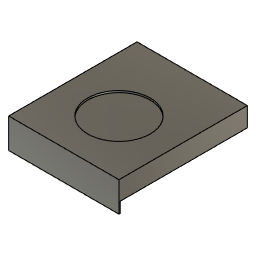
slider (Autodesk Fusion 360 design; units mm, degrees)
Autodesk Fusion 360 part; units mm, degrees
note: some values were not read from the file. Set by a fixed rule: which sketch regions a step uses.
sketch "Sketch1" plane through (0, 0, 0) normal (0, 0, 1) x (1, 0, 0) in component "Gerüst"
  line L0 (0, 0) -> (114, 0)
  line L1 (114, 0) -> (114, 114)
  line L2 (114, 114) -> (0, 114)
  line L3 (0, 114) -> (0, 0)
  circle A0 centre (7.25, 6.75) radius 2.75
  line L4 (57, 114) -> (57, 0) construction
  line L5 (0, 57) -> (114, 57) construction
  circle A1 centre (7.25, 35.25) radius 2.75
  circle A2 centre (28.75, 6.75) radius 2.75
  circle A3 centre (106.75, 6.75) radius 2.75
  circle A4 centre (85.25, 6.75) radius 2.75
  circle A5 centre (106.75, 35.25) radius 2.75
  circle A6 centre (7.25, 78.75) radius 2.75
  circle A7 centre (7.25, 107.25) radius 2.75
  circle A8 centre (28.75, 107.25) radius 2.75
  circle A9 centre (85.25, 107.25) radius 2.75
  circle A10 centre (106.75, 107.25) radius 2.75
  circle A11 centre (106.75, 78.75) radius 2.75
  line L6 (21, 100.5) -> (93, 100.5)
  line L7 (93, 100.5) -> (93, 13.5)
  line L8 (93, 13.5) -> (21, 13.5)
  line L9 (21, 13.5) -> (21, 100.5)
  line L10 (37, 114) -> (37, 131)
  line L11 (37, 131) -> (77, 131)
  line L12 (77, 131) -> (77, 114)
  line L13 (57, 131) -> (57, 114) construction
  line L14 (21, 64.5) -> (93, 64.5)
  line L15 (93, 64.5) -> (93, 49.5)
  line L16 (93, 49.5) -> (21, 49.5)
  line L17 (21, 49.5) -> (21, 64.5)
  line L18 (21, 64.5) -> (93, 49.5) construction
  line L19 (93, 64.5) -> (21, 49.5) construction
  point P0 (57, 57)
  dimension "d1" = 114
  dimension "d2" = 114
  dimension "d3" = 5.5
  dimension "d5" = 4.5
  dimension "d6" = 4
  dimension "d7" = 23
  dimension "d8" = 16
  dimension "d9" = 11
  dimension "d10" = 11
  dimension "d11" = 4
  dimension "d12" = 4
  dimension "d15" = 40
  dimension "d16" = 17
  dimension "d61" = 15
  constraint horizontal L0
  constraint vertical L1
  constraint horizontal L2
  constraint vertical L3
  constraint coincident L0.start L3.end
  constraint midpoint L2 L4.start
  constraint midpoint L0 L4.end
  constraint midpoint L3 L5.start
  constraint midpoint L1 L5.end
  constraint equal A0 A1
  constraint vertical A0.centre A1.centre
  constraint horizontal A0.centre A2.centre
  constraint equal A0 A2
  constraint symmetric A0 L4 A3
  constraint symmetric L4 A1 A5
  constraint symmetric L4 A2 A4
  constraint symmetric A0 L5 A7
  constraint symmetric L5 A1 A6
  constraint symmetric L5 A2 A8
  constraint symmetric L5 A3 A10
  constraint symmetric L5 A4 A9
  constraint symmetric L5 A5 A11
  constraint horizontal L6
  constraint vertical L7
  constraint horizontal L8
  constraint vertical L9
  constraint coincident L2 L10.start
  constraint parallel L2 L11
  constraint coincident L2 L12.end
  constraint midpoint L11 L13.start
  constraint coincident L2 L4.start
  constraint perpendicular L2 L13
  constraint collinear L4 L13
  constraint perpendicular L11 L12
  constraint perpendicular L10 L11
  constraint perpendicular L14 L15
  constraint parallel L14 L16
  constraint parallel L15 L17
  constraint horizontal L14
  constraint coincident L9 L14.start
  constraint coincident L18 P0
  constraint coincident L19 P0
  constraint midpoint L4 P0
  measures "d1" distance of L0.start L2.end
  measures "d2" distance of L0.start L0.end
  measures "d3" diameter of A0
  measures "d5" distance of L3 A0
  measures "d6" distance of L0 A0
  measures "d7" distance of A0 A1
  measures "d8" distance of A0 A2
  measures "d9" distance of A7 L9
  measures "d10" distance of A10 L7
  measures "d11" distance of A7 L6
  measures "d12" distance of A0 L8
  measures "d15" distance of L10.end L11.end
  measures "d16" distance of L2 L11
  measures "d61" distance of L14 L16
extrude "Extrude1" add sketch "Sketch1" along normal blind 5 makes body 1 in component "Gerüst"
sketch "Sketch8" plane through (0, 0, 0) normal (0, 0, -1) x (1, 0, 0) in component "Gerüst"
  circle A0 centre (106.75, -107.25) radius 2.75
  line L0 (21, -13.5) -> (93, -13.5)
  line L1 (93, -13.5) -> (93, -100.5)
  line L2 (93, -100.5) -> (21, -100.5)
  line L3 (21, -100.5) -> (21, -13.5)
  circle A1 centre (28.75, -107.25) radius 2.75
  circle A2 centre (85.25, -107.25) radius 2.75
  circle A3 centre (7.25, -107.25) radius 2.75
  circle A4 centre (85.25, -6.75) radius 2.75
  circle A5 centre (106.75, -78.75) radius 2.75
  circle A6 centre (106.75, -6.75) radius 2.75
  circle A7 centre (7.25, -78.75) radius 2.75
  circle A8 centre (28.75, -6.75) radius 2.75
  circle A9 centre (7.25, -35.25) radius 2.75
  circle A10 centre (106.75, -35.25) radius 2.75
  circle A11 centre (7.25, -6.75) radius 2.75
  line L4 (0, -114) -> (37, -114)
  line L5 (37, -114) -> (37, -131)
  line L6 (37, -131) -> (77, -131)
  line L7 (77, -131) -> (77, -114)
  line L8 (77, -114) -> (114, -114)
  line L9 (114, -114) -> (114, 0)
  line L10 (114, 0) -> (0, 0)
  line L11 (0, 0) -> (0, -114)
  line L12 (37, -131) -> (77, -131)
  line L13 (77, -131) -> (77, -117)
  line L14 (77, -117) -> (37, -117)
  line L15 (37, -117) -> (37, -131)
  dimension "d30" = 14
  constraint horizontal L12
  constraint vertical L13
  constraint horizontal L14
  constraint vertical L15
  constraint coincident L7 L13.end
  constraint coincident L5.end L6.start
  measures "d30" distance of L6.end L13.end
extrude "Extrude3" add sketch "Sketch8" along normal blind 29 contours L5 L6 L7 L12 L13 L14 L15 bodies 1 in component "Gerüst"
sketch "Sketch9" plane through (0, 0, -29) normal (0, 0, -1) x (1, 0, 0) in component "Gerüst"
  line L0 (37, -117) -> (37, -131)
  line L1 (37, -131) -> (77, -131)
  line L2 (77, -131) -> (77, -117)
  line L3 (77, -117) -> (37, -117)
  line L4 (37, -119) -> (77, -119)
  line L5 (77, -119) -> (77, -129)
  line L6 (77, -129) -> (37, -129)
  line L7 (37, -129) -> (37, -119)
  dimension "d33" = 2
  dimension "d34" = 2
  constraint horizontal L4
  constraint vertical L5
  constraint horizontal L6
  constraint vertical L7
  constraint coincident L2 L5.end
  constraint coincident L0 L4.start
  measures "d33" distance of L3 L4
  measures "d34" distance of L1 L6
extrude "Extrude4" cut sketch "Sketch9" against normal blind 6 contours L0 L2 L4 L5 L6 L7 bodies 1 in component "Gerüst"
sketch "Sketch10" plane through (0, 0, 5) normal (0, 0, 1) x (-1, 0, 0) in component "Gerüst"
  circle A0 centre (-106.75, -107.25) radius 2.75
  circle A1 centre (-85.25, -6.75) radius 2.75
  circle A2 centre (-106.75, -78.75) radius 2.75
  circle A3 centre (-7.25, -78.75) radius 2.75
  circle A4 centre (-7.25, -107.25) radius 2.75
  circle A5 centre (-28.75, -107.25) radius 2.75
  line L0 (-93, -13.5) -> (-21, -13.5)
  line L1 (-21, -13.5) -> (-21, -100.5)
  line L2 (-21, -100.5) -> (-93, -100.5)
  line L3 (-93, -100.5) -> (-93, -13.5)
  circle A6 centre (-7.25, -35.25) radius 2.75
  circle A7 centre (-85.25, -107.25) radius 2.75
  circle A8 centre (-106.75, -35.25) radius 2.75
  circle A9 centre (-28.75, -6.75) radius 2.75
  circle A10 centre (-106.75, -6.75) radius 2.75
  circle A11 centre (-7.25, -6.75) radius 2.75
  line L4 (-37, -114) -> (0, -114)
  line L5 (0, -114) -> (0, 0)
  line L6 (0, 0) -> (-114, 0)
  line L7 (-114, 0) -> (-114, -114)
  line L8 (-114, -114) -> (-77, -114)
  line L9 (-77, -114) -> (-77, -131)
  line L10 (-77, -131) -> (-37, -131)
  line L11 (-37, -131) -> (-37, -114)
  line L12 (-41, -131) -> (-73, -131)
  line L13 (-73, -131) -> (-73, -119)
  line L14 (-73, -119) -> (-41, -119)
  line L15 (-41, -119) -> (-41, -131)
  line L16 (-114, -114) -> (0, -114)
  line L17 (-77, -131) -> (-77, -114)
  line L18 (-37, -114) -> (-37, -131)
  dimension "d38" = 4
  dimension "d39" = 4
  dimension "d40" = 12
  constraint horizontal L12
  constraint vertical L13
  constraint horizontal L14
  constraint vertical L15
  constraint coincident L10 L12.start
  measures "d38" distance of L13 L17
  measures "d39" distance of L15 L18
  measures "d40" distance of L12.end L13.end
extrude "Extrude5" cut sketch "Sketch10" against normal up to surface (25 mm away) contours L10 L12 L13 L14 L15 bodies 1 in component "Gerüst"
sketch "Sketch11" plane through (0, 0, -23) normal (0, 0, -1) x (1, 0, 0) in component "Gerüst"
  line L0 (37, -129) -> (77, -129)
  line L1 (77, -129) -> (77, -119)
  line L2 (77, -119) -> (37, -119)
  line L3 (37, -119) -> (37, -129)
  circle A0 centre (57, -124) radius 1.75
  dimension "d44" = 3.5
  dimension "d45" = 5
  dimension "d46" = 20
  measures "d44" diameter of A0
  measures "d45" distance of L2 A0.centre
  measures "d46" distance of L3 A0.centre
extrude "Extrude6" cut sketch "Sketch11" against normal up to surface (3 mm away) contours A0 bodies 1 in component "Gerüst"
sketch "Sketch12" plane through (77, 0, 0) normal (1, 0, 0) x (0, 1, 0) in component "Gerüst"
  line L0 (129, -23) -> (129, -29)
  line L1 (129, -29) -> (131, -29)
  line L2 (131, -29) -> (131, 5)
  line L3 (131, 5) -> (114, 5)
  line L4 (114, 5) -> (114, 0)
  line L5 (114, 0) -> (117, 0)
  line L6 (117, 0) -> (117, -29)
  line L7 (117, -29) -> (119, -29)
  line L8 (119, -29) -> (119, -23)
  line L9 (119, -23) -> (129, -23)
  line L10 (117, -29) -> (117, 0)
  line L11 (117, 0) -> (101, 0)
  line L12 (101, 0) -> (117, -29)
  dimension "d49" = 16
  constraint coincident L6.end L7.start
  constraint coincident L5.end L6.start
  constraint perpendicular L4 L11
  measures "d49" distance of L5.end L11.end
extrude "Extrude7" add sketch "Sketch12" against normal blind 40 contours L5 L6 L10 L11 L12 bodies 1 in component "Gerüst"
extrude "Extrude8" cut sketch "Sketch12" against normal up to surface (34 mm away) from surface at -3 contours L5 L6 L10 L11 L12 bodies 1 in component "Gerüst"
sketch "Sketch13" plane through (0, 0, -29) normal (0, 0, -1) x (1, 0, 0) in component "Gerüst"
  line L0 (77, -129) -> (37, -129)
  line L1 (37, -129) -> (37, -131)
  line L2 (37, -131) -> (77, -131)
  line L3 (77, -131) -> (77, -129)
  line L4 (37, -131) -> (52, -138)
  line L5 (52, -138) -> (62, -138)
  line L6 (62, -138) -> (77, -131)
  dimension "d55" = 7
  dimension "d56" = 10
  constraint coincident L1.end L2.start
  constraint perpendicular L1 L5
  constraint coincident L2.end L3.start
  constraint equal L4 L6
  measures "d55" distance of L2 L5
  measures "d56" distance of L4.end L5.end
extrude "Extrude9" add sketch "Sketch13" against normal up to surface (9 mm away) contours L2 L4 L5 L6 bodies 1 in component "Gerüst"
chamfer "Chamfer1" distance 8 distance2 15 2 edges at (75, 131, 5) (39, 131, 5) measured on face at (96.6667, 64.25, 5) measured on face at (96.6667, 64.25, 5) on bodies 1 in component "Gerüst"
sketch "Sketch14" plane through (0, 0, 5) normal (0, 0, 1) x (-1, 0, 0) in component "Gerüst"
  line L0 (-41, -123) -> (-37, -123)
  line L1 (-37, -123) -> (-37, -114)
  line L2 (-37, -114) -> (0, -114)
  line L3 (0, -114) -> (0, 0)
  line L4 (0, 0) -> (-114, 0)
  line L5 (-114, 0) -> (-114, -114)
  line L6 (-114, -114) -> (-77, -114)
  line L7 (-77, -114) -> (-77, -123)
  line L8 (-77, -123) -> (-73, -123)
  line L9 (-73, -123) -> (-73, -119)
  line L10 (-73, -119) -> (-41, -119)
  line L11 (-41, -119) -> (-41, -123)
  line L12 (-93, -13.5) -> (-21, -13.5)
  line L13 (-21, -13.5) -> (-21, -100.5)
  line L14 (-21, -100.5) -> (-93, -100.5)
  line L15 (-93, -100.5) -> (-93, -13.5)
  circle A0 centre (-106.75, -35.25) radius 2.75
  circle A1 centre (-85.25, -6.75) radius 2.75
  circle A2 centre (-7.25, -107.25) radius 2.75
  circle A3 centre (-7.25, -6.75) radius 2.75
  circle A4 centre (-85.25, -107.25) radius 2.75
  circle A5 centre (-28.75, -107.25) radius 2.75
  circle A6 centre (-28.75, -6.75) radius 2.75
  circle A7 centre (-106.75, -6.75) radius 2.75
  circle A8 centre (-106.75, -107.25) radius 2.75
  circle A9 centre (-106.75, -78.75) radius 2.75
  circle A10 centre (-7.25, -35.25) radius 2.75
  circle A11 centre (-7.25, -78.75) radius 2.75
  circle A12 centre (-28.75, -107.25) radius 5.5
  circle A13 centre (-7.25, -107.25) radius 5.5
  circle A14 centre (-7.25, -78.75) radius 5.5
  circle A15 centre (-7.25, -35.25) radius 5.5
  circle A16 centre (-7.25, -6.75) radius 5.5
  circle A17 centre (-28.75, -6.75) radius 5.5
  circle A18 centre (-85.25, -6.75) radius 5.5
  circle A19 centre (-106.75, -6.75) radius 5.5
  circle A20 centre (-106.75, -35.25) radius 5.5
  circle A21 centre (-106.75, -78.75) radius 5.5
  circle A22 centre (-106.75, -107.25) radius 5.5
  circle A23 centre (-85.25, -107.25) radius 5.5
  line L16 (-49.5, -119) -> (-64.5, -119)
  line L17 (-64.5, -119) -> (-64.5, -100.5)
  line L18 (-64.5, -100.5) -> (-49.5, -100.5)
  line L19 (-49.5, -100.5) -> (-49.5, -119)
  line L20 (-49.5, -119) -> (-64.5, -100.5) construction
  line L21 (-49.5, -100.5) -> (-64.5, -119) construction
  line L22 (-21, -100.5) -> (-19, -100.5)
  line L23 (-19, -100.5) -> (-19, -5)
  line L24 (-19, -5) -> (-21, -5)
  line L25 (-21, -5) -> (-21, -100.5)
  line L26 (-93, -100.5) -> (-95, -100.5)
  line L27 (-95, -100.5) -> (-95, -5)
  line L28 (-95, -5) -> (-93, -5)
  line L29 (-93, -5) -> (-93, -100.5)
  point P0 (-57, -109.75)
  point P1 (-57, -124)
  dimension "d79" = 11
  dimension "d80" = 11
  dimension "d81" = 11
  dimension "d82" = 11
  dimension "d83" = 11
  dimension "d84" = 11
  dimension "d85" = 11
  dimension "d86" = 11
  dimension "d87" = 11
  dimension "d88" = 11
  dimension "d89" = 11
  dimension "d90" = 11
  dimension "d93" = 15
  dimension "d94" = 2
  dimension "d95" = 2
  dimension "d96" = 5
  constraint concentric A5 A12
  constraint concentric A2 A13
  constraint concentric A11 A14
  constraint concentric A10 A15
  constraint concentric A3 A16
  constraint concentric A6 A17
  constraint concentric A1 A18
  constraint concentric A7 A19
  constraint concentric A0 A20
  constraint concentric A9 A21
  constraint concentric A8 A22
  constraint concentric A4 A23
  constraint horizontal L16
  constraint vertical L17
  constraint horizontal L18
  constraint vertical L19
  constraint coincident L14 L17.end
  constraint coincident L10 L16.start
  constraint midpoint L21 P0
  constraint vertical P0 P1
  constraint horizontal L22
  constraint vertical L23
  constraint horizontal L24
  constraint vertical L25
  constraint coincident L13.end L14.start
  constraint horizontal L26
  constraint vertical L27
  constraint horizontal L28
  constraint vertical L29
  constraint coincident L14.end L15.start
  constraint collinear L24 L28
  measures "d79" diameter of A12
  measures "d80" diameter of A13
  measures "d81" diameter of A14
  measures "d82" diameter of A15
  measures "d83" diameter of A16
  measures "d84" diameter of A17
  measures "d85" diameter of A18
  measures "d86" diameter of A19
  measures "d87" diameter of A20
  measures "d88" diameter of A21
  measures "d89" diameter of A22
  measures "d90" diameter of A23
  measures "d93" distance of L16.start L16.end
  measures "d94" distance of L13.end L22.end
  measures "d95" distance of L14.end L26.end
  measures "d96" distance of L4 L24
extrude "Extrude11" cut sketch "Sketch14" against normal up to surface (3 mm away) contours A12 | A13 | A14 | A15 | A16 | A17 | A18 | A19 | A20 | A21 | A22 | A23 bodies 1 in component "Gerüst"
extrude "Extrude12" add sketch "Sketch14" along normal blind 8 contours L13 L22 L23 L24 L25 | L15 L26 L27 L28 L29 bodies 1 in component "Gerüst"
extrude "Extrude13" add sketch "Sketch14" along normal blind 4 contours L10 L14 L16 L17 L18 L19 bodies 1 in component "Gerüst"
chamfer "Chamfer2" distance 18.5 distance2 3 1 edges at (57, 100.5, 9) measured on face at (59.5, 106.6667, 9) on bodies 1 in component "Gerüst"
chamfer "Chamfer3" distance 8 angle 45 2 edges at (94, 5, 13) (20, 5, 13) on bodies 1 in component "Gerüst"
sketch "Sketch15" plane through (95, 0, 0) normal (1, 0, 0) x (0, 1, 0) in component "Gerüst"
  line L0 (13, 13) -> (5, 5)
  line L1 (5, 5) -> (100.5, 5)
  line L2 (100.5, 5) -> (100.5, 13)
  line L3 (100.5, 13) -> (13, 13)
  line L4 (13, 13) -> (100.5, 13)
  line L5 (100.5, 13) -> (100.5, 11)
  line L6 (100.5, 11) -> (13, 11)
  line L7 (13, 11) -> (13, 13)
  dimension "d104" = 2
  constraint horizontal L4
  constraint vertical L5
  constraint horizontal L6
  constraint vertical L7
  constraint coincident L2 L5.end
  constraint coincident L0.start L3.end
  measures "d104" distance of L2.end L5.end
extrude "Extrude14" add sketch "Sketch15" along normal blind 4 contours L2 L3 L4 L5 L6 L7 bodies 1 in component "Gerüst"
extrude "Extrude15" add sketch "Sketch15" against normal blind 4 from surface at -76 contours L2 L3 L4 L5 L6 L7 bodies 1 in component "Gerüst"
fillet "Fillet1" [suppressed] in component "Gerüst"
extrude "Extrude16" add sketch "Sketch1" along normal blind 3 contours L7 L9 L14 L15 L16 L17 bodies 1 in component "Gerüst"
sketch "Sketch16" plane through (0, 0, 0) normal (0, 0, -1) x (1, 0, 0) in component "Gerüst"
  line L0 (21, -49.5) -> (21, -13.5)
  line L1 (21, -13.5) -> (93, -13.5)
  line L2 (93, -13.5) -> (93, -49.5)
  line L3 (93, -49.5) -> (21, -49.5)
  line L4 (77, -101) -> (77, -114)
  line L5 (77, -114) -> (114, -114)
  line L6 (114, -114) -> (114, 0)
  line L7 (114, 0) -> (0, 0)
  line L8 (0, 0) -> (0, -114)
  line L9 (0, -114) -> (37, -114)
  line L10 (37, -114) -> (37, -101)
  line L11 (37, -101) -> (40, -101)
  line L12 (40, -101) -> (40, -117)
  line L13 (40, -117) -> (74, -117)
  line L14 (74, -117) -> (74, -101)
  line L15 (74, -101) -> (77, -101)
  circle A0 centre (106.75, -35.25) radius 2.75
  circle A1 centre (7.25, -78.75) radius 2.75
  circle A2 centre (106.75, -107.25) radius 2.75
  circle A3 centre (85.25, -6.75) radius 2.75
  circle A4 centre (28.75, -6.75) radius 2.75
  circle A5 centre (28.75, -107.25) radius 2.75
  circle A6 centre (7.25, -6.75) radius 2.75
  circle A7 centre (106.75, -6.75) radius 2.75
  line L16 (21, -64.5) -> (93, -64.5)
  line L17 (93, -64.5) -> (93, -100.5)
  line L18 (93, -100.5) -> (21, -100.5)
  line L19 (21, -100.5) -> (21, -64.5)
  circle A8 centre (106.75, -78.75) radius 2.75
  circle A9 centre (7.25, -35.25) radius 2.75
  circle A10 centre (7.25, -107.25) radius 2.75
  circle A11 centre (85.25, -107.25) radius 2.75
  line L20 (25, -51.5) -> (27, -51.5)
  line L21 (27, -62.5) -> (25, -62.5)
  line L22 (25, -62.5) -> (25, -51.5)
  line L23 (57, 0) -> (57, -117) construction
  line L24 (27, -56) -> (47, -56)
  line L25 (47, -56) -> (47, -58)
  line L26 (47, -58) -> (27, -58)
  line L27 (27, -51.5) -> (27, -56)
  line L28 (27, -58) -> (27, -62.5)
  line L29 (87, -56) -> (67, -56)
  line L30 (67, -56) -> (67, -58)
  line L31 (67, -58) -> (87, -58)
  line L32 (87, -58) -> (87, -62.5)
  line L33 (87, -62.5) -> (89, -62.5)
  line L34 (89, -62.5) -> (89, -51.5)
  line L35 (87, -51.5) -> (87, -56)
  line L36 (89, -51.5) -> (87, -51.5)
  dimension "d113" = 25
  dimension "d114" = 2
  dimension "d115" = 2
  dimension "d116" = 2
  dimension "d117" = 20
  dimension "d118" = 2
  constraint horizontal L20
  constraint vertical L27
  constraint horizontal L21
  constraint vertical L22
  constraint midpoint L7 L23.start
  constraint midpoint L13 L23.end
  constraint horizontal L24
  constraint vertical L25
  constraint horizontal L26
  constraint collinear L27 L28
  constraint equal L27 L28
  constraint symmetric L20.start L23 L34.end
  constraint symmetric L20.end L23 L35.start
  constraint symmetric L21.start L23 L32.end
  constraint symmetric L21.end L23 L33.end
  constraint symmetric L23 L24.start L29.start
  constraint symmetric L23 L24.end L29.end
  constraint symmetric L23 L25.end L30.end
  constraint symmetric L23 L26.end L31.end
  measures "d113" distance of L8 L22
  measures "d114" distance of L20.start L20.end
  measures "d115" distance of L3 L20
  measures "d116" distance of L16 L21
  measures "d117" distance of L24.start L24.end
  measures "d118" distance of L24.end L25.end
extrude "Extrude17" add sketch "Sketch16" along normal blind 40 contours L20 L21 L22 L24 L25 L26 L27 L28 | L29 L30 L31 L32 L33 L34 L35 L36 bodies 1 in component "Gerüst"
chamfer "Chamfer4" distance 20 distance2 40 2 edges at (47, 57, -40) (67, 57, -40) measured on face at (25.6667, 56.6667, -40) measured on face at (88.3333, 56.6667, -40) on bodies 1 in component "Gerüst"
fillet "Fillet2" radius 3 4 edges at (88, 51.5, -40) (88, 62.5, -40) (26, 51.5, -40) (26, 62.5, -40) on bodies 1 in component "Gerüst"
sketch "Sketch1 (2)" plane through (0, 0, 13) normal (0, 0, 1) x (-1, 0, 0) in component "Blende"
  line L0 (-99, -100.5) -> (-93, -100.5)
  line L1 (-93, -100.5) -> (-93, -13)
  line L2 (-93, -13) -> (-95, -13)
  line L3 (-114, 0) -> (-114, -114)
  line L4 (0, -114) -> (0, 0)
  line L5 (0, 0) -> (-114, 0)
  line L6 (-52, -138) -> (-62, -138)
  line L7 (-99.3, -13) -> (-101.3, -13)
  line L8 (-101.3, -13) -> (-101.3, -100.5)
  line L9 (-101.3, -100.5) -> (-99.3, -100.5)
  line L10 (-99.3, -100.5) -> (-99.3, -13)
  line L11 (-93, -13.5) -> (-21, -13.5)
  line L12 (-95, -13) -> (-99, -13)
  line L13 (-99, -13) -> (-99, -100.5)
  line L14 (-57, -138) -> (-57, 5) construction
  line L15 (-12.7, -13) -> (-12.7, -100.5)
  line L16 (-12.7, -100.5) -> (-14.7, -100.5)
  line L17 (-14.7, -100.5) -> (-14.7, -13)
  line L18 (-14.7, -13) -> (-12.7, -13)
  dimension "d127" = 0.3
  dimension "d129" = 2
  constraint horizontal L7
  constraint vertical L8
  constraint horizontal L9
  constraint vertical L10
  constraint collinear L7 L12
  constraint collinear L0 L9
  constraint symmetric L7.start L14 L17.end
  constraint symmetric L7.end L14 L15.start
  constraint symmetric L8.end L14 L15.end
  constraint symmetric L9.end L14 L16.end
  measures "d127" distance of L10 L13
  measures "d129" distance of L8.end L9.end
extrude "Extrude1'" add sketch "Sketch1 (2)" along normal blind 0.3 and the other way up to surface (4.3 mm away) separate body contours L7 L8 L9 L10 | L15 L16 L17 L18 makes body 2 at (99.3, 71.3333, 11.7667) makes body 3 at (12.7, 42.1667, 11.7667) in component "Blende"
sketch "Sketch3" plane through (99.3, 0, 0) normal (-1, 0, 0) x (0, -1, 0) in component "Blende"
  line L0 (-13, 8.7) -> (-13, 13.3)
  line L1 (-13, 13.3) -> (-100.5, 13.3)
  line L2 (-100.5, 13.3) -> (-100.5, 8.7)
  line L3 (-100.5, 8.7) -> (-13, 8.7)
  line L4 (-13, 8.7) -> (-100.5, 8.7)
  line L5 (-100.5, 8.7) -> (-100.5, 10.7)
  line L6 (-100.5, 10.7) -> (-13, 10.7)
  line L7 (-13, 10.7) -> (-13, 8.7)
  dimension "d138" = 2
  constraint horizontal L4
  constraint vertical L5
  constraint horizontal L6
  constraint vertical L7
  constraint coincident L0.start L3.end
  measures "d138" distance of L2.end L5.end
extrude "Extrude3'" add sketch "Sketch3" along normal blind 3.5 contours L0 L2 L3 L4 L5 L6 L7 bodies 2 in component "Blende"
extrude "Extrude4'" add sketch "Sketch3" against normal blind 3.5 from surface at 84.6 contours L0 L2 L3 L4 L5 L6 L7 bodies 3 in component "Blende"
sketch "Sketch4" plane through (0, 0, 13.3) normal (0, 0, 1) x (-1, 0, 0) in component "Blende"
  line L0 (-99.3, -100.5) -> (-99.3, -13)
  line L1 (-99.3, -13) -> (-101.3, -13)
  line L2 (-101.3, -13) -> (-101.3, -100.5)
  line L3 (-101.3, -100.5) -> (-99.3, -100.5)
  line L4 (4, -138) -> (-118, -138)
  line L5 (-118, -138) -> (-118, 4)
  line L6 (-118, 4) -> (4, 4)
  line L7 (4, 4) -> (4, -138)
  line L8 (0, 0) -> (-114, 0)
  line L9 (0, -114) -> (0, 0)
  line L10 (-114, 0) -> (-114, -114)
  line L11 (-52, -138) -> (-62, -138)
  dimension "d144" = 4
  dimension "d145" = 4
  dimension "d146" = 4
  constraint horizontal L4
  constraint vertical L5
  constraint horizontal L6
  constraint vertical L7
  constraint collinear L4 L11
  measures "d144" distance of L6 L8
  measures "d145" distance of L7 L9
  measures "d146" distance of L5 L10
extrude "Extrude5'" add sketch "Sketch4" along normal blind 3 contours L0 L1 L2 L3 | L4 L5 L6 L7 L11 bodies 2 3 in component "Blende"
sketch "Sketch5" plane through (0, 0, 5) normal (0, 0, 1) x (-1, 0, 0) in component "Blende"
  line L0 (-64.5, -119) -> (-64.5, -100.5)
  line L1 (-64.5, -100.5) -> (-93, -100.5)
  line L2 (-93, -100.5) -> (-95, -100.5)
  line L3 (-95, -100.5) -> (-95, -5)
  line L4 (-95, -5) -> (-93, -5)
  line L5 (-93, -5) -> (-93, -13.5)
  line L6 (-93, -13.5) -> (-21, -13.5)
  line L7 (-21, -13.5) -> (-21, -5)
  line L8 (-21, -5) -> (-19, -5)
  line L9 (-19, -5) -> (-19, -100.5)
  line L10 (-19, -100.5) -> (-21, -100.5)
  line L11 (-21, -100.5) -> (-49.5, -100.5)
  line L12 (-49.5, -100.5) -> (-49.5, -119)
  line L13 (-49.5, -119) -> (-41, -119)
  line L14 (-41, -119) -> (-41, -123)
  line L15 (-41, -123) -> (-37, -123)
  line L16 (-37, -123) -> (-37, -114)
  line L17 (-37, -114) -> (0, -114)
  line L18 (0, -114) -> (0, 0)
  line L19 (0, 0) -> (-114, 0)
  line L20 (-114, 0) -> (-114, -114)
  line L21 (-114, -114) -> (-77, -114)
  line L22 (-77, -114) -> (-77, -123)
  line L23 (-77, -123) -> (-73, -123)
  line L24 (-73, -123) -> (-73, -119)
  line L25 (-73, -119) -> (-64.5, -119)
  circle A0 centre (-106.75, -6.75) radius 5.5
  circle A1 centre (-85.25, -107.25) radius 5.5
  circle A2 centre (-7.25, -35.25) radius 5.5
  circle A3 centre (-7.25, -78.75) radius 5.5
  circle A4 centre (-106.75, -107.25) radius 5.5
  circle A5 centre (-85.25, -6.75) radius 5.5
  circle A6 centre (-106.75, -35.25) radius 5.5
  circle A7 centre (-28.75, -107.25) radius 5.5
  circle A8 centre (-7.25, -6.75) radius 5.5
  circle A9 centre (-7.25, -107.25) radius 5.5
  circle A10 centre (-106.75, -78.75) radius 5.5
  circle A11 centre (-28.75, -6.75) radius 5.5
  line L26 (-49.25, -119.35) -> (-64.75, -119.35)
  line L27 (-64.75, -119.35) -> (-64.75, -100.25)
  line L28 (-64.75, -100.25) -> (-49.25, -100.25)
  line L29 (-49.25, -100.25) -> (-49.25, -119.35)
  line L30 (-49.5, -100.5) -> (-64.5, -100.5)
  line L31 (-64.5, -119) -> (-49.5, -119)
  line L32 (-44.25, -129.35) -> (-69.75, -129.35)
  line L33 (-69.75, -129.35) -> (-69.75, -95.25)
  line L34 (-69.75, -95.25) -> (-44.25, -95.25)
  line L35 (-44.25, -95.25) -> (-44.25, -129.35)
  dimension "d149" = 0.25
  dimension "d150" = 0.35
  dimension "d151" = 0.25
  dimension "d152" = 0.25
  dimension "d153" = 5
  dimension "d154" = 5
  dimension "d155" = 10
  dimension "d156" = 5
  constraint horizontal L26
  constraint vertical L27
  constraint horizontal L28
  constraint vertical L29
  constraint horizontal L32
  constraint vertical L33
  constraint horizontal L34
  constraint vertical L35
  measures "d149" distance of L28 L30
  measures "d150" distance of L26 L31
  measures "d151" distance of L12 L29
  measures "d152" distance of L0 L27
  measures "d153" distance of L27 L33
  measures "d154" distance of L29 L35
  measures "d155" distance of L26 L32
  measures "d156" distance of L28 L34
extrude "Extrude6'" add sketch "Sketch5" along normal blind 1.5 from surface at 1.3 separate body contours L13 L25 L26 L27 L29 L32 L33 L35 | L1 L25 L27 L33 | L1 L11 L27 L28 L29 L33 L34 L35 | L11 L13 L29 L35 makes body 4 in component "Blende"
sketch "Sketch6" plane through (0, 0, 7.8) normal (0, 0, 1) x (-1, 0, 0) in component "Blende"
  line L0 (-64.75, -100.25) -> (-49.25, -100.25)
  line L1 (-49.25, -100.25) -> (-49.25, -119.35)
  line L2 (-49.25, -119.35) -> (-64.75, -119.35)
  line L3 (-64.75, -119.35) -> (-64.75, -100.25)
  line L4 (-44.25, -95.25) -> (-69.75, -95.25)
  line L5 (-69.75, -95.25) -> (-69.75, -129.35)
  line L6 (-69.75, -129.35) -> (-44.25, -129.35)
  line L7 (-44.25, -129.35) -> (-44.25, -95.25)
  line L8 (-44.25, -95.25) -> (-69.75, -95.25)
  line L9 (-69.75, -95.25) -> (-69.75, -98.25)
  line L10 (-69.75, -98.25) -> (-44.25, -98.25)
  line L11 (-44.25, -98.25) -> (-44.25, -95.25)
  dimension "d160" = 3
  constraint horizontal L8
  constraint vertical L9
  constraint horizontal L10
  constraint vertical L11
  constraint coincident L4.start L7.end
  constraint collinear L5 L9
  measures "d160" distance of L4.start L10.end
extrude "Extrude7'" add sketch "Sketch6" along normal up to surface (5.5 mm away) contours L4 L5 L7 L8 L9 L10 L11 bodies 2 4 in component "Blende"
sketch "Sketch7" plane through (0, 13, 0) normal (0, -1, 0) x (1, 0, 0) in component "Blende"
  line L0 (101.3, 8.7) -> (101.3, 13.3)
  line L1 (101.3, 13.3) -> (99.3, 13.3)
  line L2 (99.3, 13.3) -> (99.3, 10.7)
  line L3 (99.3, 10.7) -> (95.8, 10.7)
  line L4 (95.8, 10.7) -> (95.8, 8.7)
  line L5 (95.8, 8.7) -> (101.3, 8.7)
  line L6 (101.3, 8.7) -> (95.8, 8.7)
  line L7 (95.8, 8.7) -> (95.8, 13.3)
  line L8 (95.8, 13.3) -> (101.3, 13.3)
  line L9 (101.3, 13.3) -> (101.3, 8.7)
  line L10 (118, 13.3) -> (-4, 13.3)
  line L11 (57, 13.3) -> (57, 3.3) construction
  line L12 (12.7, 8.7) -> (18.2, 8.7)
  line L13 (12.7, 13.3) -> (12.7, 8.7)
  line L14 (18.2, 13.3) -> (12.7, 13.3)
  line L15 (18.2, 8.7) -> (18.2, 13.3)
  dimension "d163" = 10
  constraint horizontal L6
  constraint vertical L7
  constraint horizontal L8
  constraint vertical L9
  constraint coincident L4 L7.end
  constraint coincident L0.start L5.end
  constraint collinear L8 L10
  constraint midpoint L10 L11.start
  constraint perpendicular L10 L11
  constraint symmetric L0.start L11 L12.start
  constraint symmetric L4.end L11 L12.end
  constraint symmetric L7.end L11 L14.start
  constraint symmetric L0.end L11 L13.start
  measures "d163" distance of L11.start L11.end
extrude "Extrude8'" add sketch "Sketch7" along normal blind 2 bodies 2 in component "Blende"
sketch "Sketch8 (2)" plane through (0, 0, 16.3) normal (0, 0, 1) x (-1, 0, 0) in component "Blende"
  line L0 (-118, -138) -> (4, -138)
  line L1 (4, -138) -> (4, 4)
  line L2 (4, 4) -> (-118, 4)
  line L3 (-118, 4) -> (-118, -138)
  circle A0 centre (-57, -57) radius 35.5
  line L4 (-57, -114) -> (-57, 0)
  line L5 (-93, -100.5) -> (-93, -13.5)
  circle A1 centre (-57, -57) radius 34.5
  dimension "d167" = 0.5
  dimension "d175" = 70
  dimension "d189" = -1
  constraint midpoint A0.centre L4
  measures "d167" distance of A0 L5
extrude "Extrude9'" add sketch "Sketch8 (2)" against normal blind 2 from surface at -3 contours A0 L4 A1 | A0 L4 A1 | L4 A1 | L4 A1 bodies 2 in component "Blende"
extrude "Extrude11'" cut sketch "Sketch8 (2)" against normal blind 2 contours L4 A1 | L4 A1 bodies 2 in component "Blende"
sketch "Sketch9 (2)" plane through (0, 0, 13.3) normal (0, 0, -1) x (1, 0, 0) in component "Blende"
  line L0 (-4, -138) -> (118, -138)
  line L1 (118, -138) -> (118, 4)
  line L2 (118, 4) -> (-4, 4)
  line L3 (-4, 4) -> (-4, -138)
  line L4 (12.7, -100.5) -> (12.7, -11)
  line L5 (12.7, -11) -> (18.2, -11)
  line L6 (18.2, -11) -> (18.2, -13)
  line L7 (18.2, -13) -> (14.7, -13)
  line L8 (14.7, -13) -> (14.7, -100.5)
  line L9 (14.7, -100.5) -> (12.7, -100.5)
  line L10 (44.25, -98.25) -> (44.25, -95.25)
  line L11 (44.25, -95.25) -> (69.75, -95.25)
  line L12 (69.75, -95.25) -> (69.75, -98.25)
  line L13 (69.75, -98.25) -> (44.25, -98.25)
  line L14 (101.3, -11) -> (101.3, -100.5)
  line L15 (101.3, -100.5) -> (99.3, -100.5)
  line L16 (99.3, -100.5) -> (99.3, -13)
  line L17 (99.3, -13) -> (95.8, -13)
  line L18 (95.8, -13) -> (95.8, -11)
  line L19 (95.8, -11) -> (101.3, -11)
  line L20 (-4, 4) -> (118, 4)
  line L21 (118, 4) -> (118, 2.5)
  line L22 (118, 2.5) -> (-4, 2.5)
  line L23 (-4, 2.5) -> (-4, 4)
  line L24 (-4, -138) -> (-2.5, -138)
  line L25 (-2.5, -138) -> (-2.5, 2.5)
  line L26 (-2.5, 2.5) -> (-4, 2.5)
  line L27 (-4, 2.5) -> (-4, -138)
  line L28 (118, -138) -> (116.5, -138)
  line L29 (116.5, -138) -> (116.5, 2.5)
  line L30 (116.5, 2.5) -> (118, 2.5)
  line L31 (118, 2.5) -> (118, -138)
  circle A0 centre (57, -57) radius 35.5
  dimension "d181" = 1.5
  dimension "d182" = 1.5
  constraint horizontal L20
  constraint vertical L21
  constraint horizontal L22
  constraint vertical L23
  constraint coincident L1 L21.end
  constraint coincident L2.end L3.start
  constraint horizontal L24
  constraint vertical L25
  constraint horizontal L26
  constraint vertical L27
  constraint coincident L22 L25.end
  constraint coincident L0.start L3.end
  constraint horizontal L28
  constraint vertical L29
  constraint horizontal L30
  constraint vertical L31
  constraint coincident L22 L29.end
  constraint coincident L0.end L1.start
  constraint equal L24 L28
  measures "d181" distance of L20 L22
  measures "d182" distance of L25 L27
extrude "Extrude12'" add sketch "Sketch9 (2)" along normal blind 30 contours L1 L2 L3 L20 L21 L22 L23 L26 L30 bodies 2 in component "Blende"
extrude "Extrude13'" add sketch "Sketch9 (2)" along normal up to surface (18.3 mm away) contours L0 L3 L22 L24 L25 L26 L27 | L0 L1 L22 L28 L29 L30 L31 bodies 2 in component "Blende"
component "Gerüst" placed x (1, 0, 0) y (0, 1, 0) z (0, 0, 1) at (0, 0, 0)
component "Blende" placed x (1, 0, 0) y (0, 1, 0) z (0, 0, 1) at (0, 0, 0)
